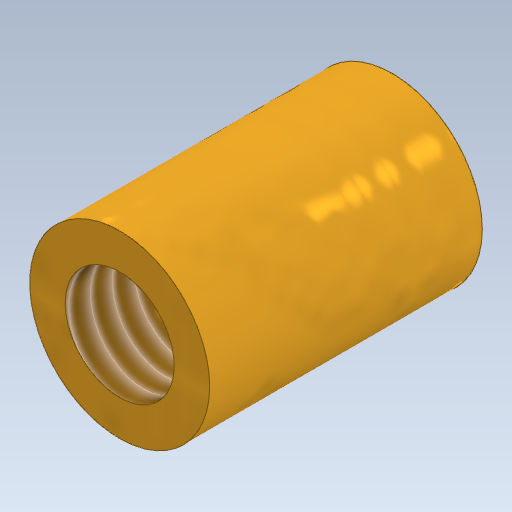
# Autodesk Inventor part: BRM2-4.1
Saved by Autodesk Inventor 2020.4 (Build 244396000, 396)
## iProperties
Part Number: BRM2-4.1
Material: 真鍮
Document SubType Name: Modeling
Designer: Masato Kubotera
Density: 5.54386 g/cm^3
Appearance: 溶接 - 真鍮
Catalog Web Link: https://jp.misumi-ec.com/vona2/detail/221005351346/?HissuCode=BRM2-4.1
Description: ReadyMade
Mass: 0.15 g
Surface Area: 0.94075 cm^2
Volume: 0.027057 cm^3
Author: Masato Kubotera
Autodesk Inventor part; units mm, degrees
ref_plane "YZ Plane" through (0, 0, 0) normal (1, 0, 0) x (0, 1, 0)
ref_plane "XZ Plane" through (0, 0, 0) normal (0, 1, 0) x (-1, 0, 0)
ref_plane "XY Plane" through (0, 0, 0) normal (0, 0, 1) x (1, 0, 0)
sketch "スケッチ1" plane through (0, 0, 0) normal (0, 0, 1) x (1, 0, 0)
  circle A0 centre (0, 0) radius 1.65
  circle A1 centre (0, 0) radius 1
  dimension "d0" = 3.3
  dimension "d1" = 2
  constraints: 2 centre point, 2 coincident
  measures "d0" diameter of A0
  measures "d1" diameter of A1
extrude "押し出し1" add sketch "スケッチ1" along normal blind 5
thread "ねじ1" size "M2x0.4" class "6H" standard "ANSI Metric M Profile" full length
